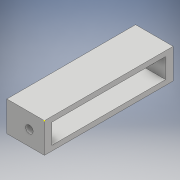
# Autodesk Inventor part: pilarSoporteLED
Saved by Autodesk Inventor 2017 (Build 210142000, 142)
## iProperties
Part Number: pilarSoporteLED
Material: Genérico
Document SubType Name: Modeling
Designer: Roberto
Density: 1 g/cm^3
Appearance: Valor por defecto
Author: Roberto
Autodesk Inventor part; units mm, degrees
ref_plane "YZ Plane" through (0, 0, 0) normal (1, 0, 0) x (0, 1, 0)
ref_plane "XZ Plane" through (0, 0, 0) normal (0, 1, 0) x (-1, 0, 0)
ref_plane "XY Plane" through (0, 0, 0) normal (0, 0, 1) x (1, 0, 0)
sketch "Boceto1" plane through (0, 0, 0) normal (0, 1, 0) x (-1, 0, 0)
  line L0 (0, 0) -> (0, -1.2)
  line L1 (0, -1.2) -> (1.2, -1.2)
  line L2 (1.2, -1) -> (1.2, -0.2)
  circle A0 centre (0.9, -0.6) radius 0.15
  circle A1 centre (0.3, -0.6) radius 0.15
  line L3 (0, 0) -> (1.5, 0)
  line L4 (1.5, 0) -> (1.5, -1.2)
  line L5 (1.5, -1.2) -> (0, -1.2)
  line L6 (0, 0) -> (0, -0.2)
  line L7 (0, -0.2) -> (1.2, -0.2)
  line L8 (0, -1.2) -> (0, -1)
  line L9 (0, -1) -> (1.2, -1)
  line L10 (0, 0) -> (0, -0.2)
  line L11 (0, -1) -> (0, -1.2)
  dimension "d0" = 1.2
  dimension "d1" = 1.2
  dimension "d3" = 0.3
  dimension "d4" = 0.3
  dimension "d5" = 1.5
  dimension "d6" = 1.2
  dimension "d7" = 0.2
  dimension "d8" = 0.2
  constraints: 24 end point, 5 perpendicular, 3 vertical, 2 centre point, 2 point on line, 1 horizontal
  measures "d0" distance of L0.start L0.end
  measures "d1" distance of L0.end L1.end
  measures "d3" diameter of A0
  measures "d4" diameter of A1
  measures "d5" distance of L0.start L3.end
  measures "d6" distance of L3.end L4.end
  measures "d7" distance of L0.start L6.end
  measures "d8" distance of L0.end L8.end
extrude "Extrusión1" add sketch "Boceto1" along normal blind 5.1401 contours L3 L4 L5 L1 L0 L9 L2 L7
sketch "Boceto5" plane through (0, 5.1401, 0) normal (0, 1, 0) x (1, 0, 0)
  line L0 (0, 0.2) -> (0, 1)
  line L1 (-1.2, 1) -> (0, 1)
  line L2 (-1.2, 0.2) -> (0, 0.2)
  circle A0 centre (-0.6, 0.6) radius 0.15
  line L3 (0, 0.2) -> (-1.2, 0.2) projected
  line L4 (-1.2, 1) -> (0, 1) projected
  line L5 (-1.2, 0.2) -> (-1.2, 1) projected
  line L6 (0, 0) -> (0, 0.2) projected
  line L7 (0, 1) -> (0, 0.2)
  constraints: 8 end point, 2 perpendicular, 1 centre point, 1 vertical
extrude "Extrusión4" add sketch "Boceto5" against normal blind 0.3
sketch "Boceto6" plane through (0, 0, 0) normal (0, -1, 0) x (1, 0, 0)
  circle A0 centre (-0.6, -0.6) radius 0.15 projected
  line L0 (-1.2, -0.2) -> (0, -0.2) projected
  line L1 (-1.2, -1) -> (-1.2, -0.2) projected
  line L2 (0, -1) -> (-1.2, -1) projected
  line L3 (0, -1) -> (0, -0.2) projected
  point P0 (0, 0)
extrude "Extrusión5" add sketch "Boceto6" against normal blind 0.3
sketch "Boceto8" plane through (-1.5, 0, 0) normal (0, 0, 1) x (1, 0, 0)
  point P0 (1.5, 0)
